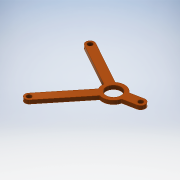
# Autodesk Inventor part: Pok Mk3 Base
Saved by Autodesk Inventor 2018.2 (Build 222227000, 227)
## iProperties
Created: 2018-02-12
Part Number: Pok Mk3 Base
Material: ABS Plastic
Document SubType Name: Modeling
Designer: Moochster
Density: 1.06 g/cm^3
Appearance: Smooth - Light Orange
Author: Moochster
Autodesk Inventor part; units mm, degrees
ref_plane "YZ Plane" through (0, 0, 0) normal (1, 0, 0) x (0, 1, 0)
ref_plane "XZ Plane" through (0, 0, 0) normal (0, 1, 0) x (-1, 0, 0)
ref_plane "XY Plane" through (0, 0, 0) normal (0, 0, 1) x (1, 0, 0)
sketch "Sketch1" plane through (0, 0, 0) normal (0, 0, 1) x (1, 0, 0)
  circle A0 centre (0, 0) radius 8.0875 projected
  circle A1 centre (24.5358, 4.7954) radius 2.5 projected
  circle A2 centre (-56.8826, 31.4543) radius 2.5 projected
  circle A3 centre (-40.854, -50.5564) radius 2.5 projected
  arc A4 (-7.5575, 9.3212) -> (-11.9127, 1.4452) centre (0, 0) ccw
  line L0 (11.6652, -2.8147) -> (25.4949, -0.1118)
  arc A5 (25.4949, -0.1118) -> (23.5767, 9.7025) centre (24.5358, 4.7954) ccw
  line L1 (23.5767, 9.7025) -> (9.7471, 6.9996)
  line L2 (0, 0) -> (24.5358, 4.7954) construction
  line L3 (0, 0) -> (-56.8826, 31.4543) construction
  line L4 (-7.5575, 9.3212) -> (-54.705, 35.3923)
  arc A6 (-54.705, 35.3923) -> (-59.0602, 27.5163) centre (-56.8826, 31.4543) ccw
  line L5 (-59.0602, 27.5163) -> (-11.9127, 1.4452)
  arc A7 (9.7471, 6.9996) -> (-7.5575, 9.3212) centre (0, 0) ccw
  arc A8 (-11.9127, 1.4452) -> (-10.4919, -5.824) centre (0, 0) ccw
  line L6 (-3.4918, -11.4807) -> (-37.3539, -53.3848)
  arc A9 (-44.3541, -47.7281) -> (-37.3539, -53.3848) centre (-40.854, -50.5564) ccw
  line L7 (-44.3541, -47.7281) -> (-10.4919, -5.824)
  arc A10 (-3.4918, -11.4807) -> (9.7471, 6.9996) centre (0, 0) ccw
  arc A11 (-10.4919, -5.824) -> (-3.4918, -11.4807) centre (0, 0) ccw
  point P0 (0, 0)
  dimension "d0" = 24
  dimension "d1" = 2.5
  dimension "d2" = 2
  constraints: 19 point on circle, 16 end point, 8 centre point, 5 symmetric about line, 4 parallel, 4 tangent, 2 concentric, 1 coincident, 1 other
  measures "d0" diameter of A4
  measures "d1" radial gap between concentric circles of A1 A5
  measures "d2" radial gap between concentric circles of A2 A6
extrude "Extrusion1" add sketch "Sketch1" against normal blind 4
body "Solid1"
